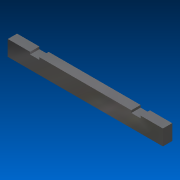
# Autodesk Inventor part: spacer 1
Saved by Autodesk Inventor 2012 (Build 160160000, 160)
## iProperties
Created: 2012-07-02
Part Number: spacer 1
Material: Default
Document SubType Name: Modeling
Designer: Hemant
Density: 1 g/cm^3
Author: Hemant
Autodesk Inventor part; units mm, degrees
ref_plane "YZ Plane" through (0, 0, 0) normal (1, 0, 0) x (0, 1, 0)
ref_plane "XZ Plane" through (0, 0, 0) normal (0, 1, 0) x (-1, 0, 0)
ref_plane "XY Plane" through (0, 0, 0) normal (0, 0, 1) x (1, 0, 0)
sketch "Sketch1" plane through (0, 0, 0) normal (0, 0, 1) x (1, 0, 0)
  line L0 (0, 0) -> (424.18, 0)
  line L1 (424.18, 0) -> (424.18, 42.3672)
  line L2 (424.18, 42.3672) -> (0, 42.3672)
  line L3 (0, 42.3672) -> (0, 0)
  dimension "d0" = 42.3672
  dimension "d1" = 424.18
  constraints: 8 end point, 2 parallel, 1 horizontal, 1 perpendicular
  measures "d0" distance between parallel lines of L2 L0
  measures "d1" distance between parallel lines of L1 L3
extrude "Extrusion1" add sketch "Sketch1" against normal blind 25.4
sketch "Sketch2" plane through (0, 0, 0) normal (0, 0, 1) x (1, 0, 0)
  line L0 (424.18, 0) -> (424.18, 42.3672) projected
  line L1 (424.18, 42.3672) -> (0, 42.3672) projected
  line L2 (0, 42.3672) -> (0, 0) projected
  line L3 (60.96, 42.3672) -> (86.36, 42.3672)
  line L4 (86.36, 42.3672) -> (86.36, 36.0172)
  line L5 (86.36, 36.0172) -> (60.96, 36.0172)
  line L6 (60.96, 36.0172) -> (60.96, 42.3672)
  line L7 (363.22, 42.3672) -> (337.82, 42.3672)
  line L8 (337.82, 42.3672) -> (337.82, 36.0172)
  line L9 (337.82, 36.0172) -> (363.22, 36.0172)
  line L10 (363.22, 36.0172) -> (363.22, 42.3672)
  dimension "d4" = 6.35
  dimension "d5" = 25.4
  dimension "d6" = 60.96
  dimension "d7" = 60.96
  dimension "d8" = 25.4
  dimension "d9" = 6.35
  constraints: 16 end point, 4 parallel, 2 horizontal, 2 perpendicular, 2 point on line
  measures "d4" distance between parallel lines of L1 L5
  measures "d5" distance between parallel lines of L4 L6
  measures "d6" distance between parallel lines of L6 L2
  measures "d7" distance between parallel lines of L10 L0
  measures "d8" distance between parallel lines of L8 L10
  measures "d9" distance between parallel lines of L1 L9
extrude "Extrusion2" cut sketch "Sketch2" against normal blind 45.72
body "Solid1"
